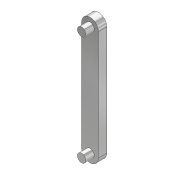
# Autodesk Inventor part: Eslabón 3
Saved by Autodesk Inventor 2021 (Build 250183000, 183)
## iProperties
Created: 2021-10-18
Part Number: Eslabón 3
Material: Steel
Document SubType Name: Modeling
Designer: Usuario
Density: 7.85 g/cm^3
Appearance: Aluminum - Dark
Author: Usuario
Autodesk Inventor part; units mm, degrees
ref_plane "YZ Plane" through (0, 0, 0) normal (1, 0, 0) x (0, 1, 0)
ref_plane "XZ Plane" through (0, 0, 0) normal (0, 1, 0) x (-1, 0, 0)
ref_plane "XY Plane" through (0, 0, 0) normal (0, 0, 1) x (1, 0, 0)
sketch "Sketch1" plane through (0, 0, 0) normal (0, 0, 1) x (1, 0, 0)
  circle A0 centre (0, 0) radius 5
  circle A1 centre (0, 130) radius 5
  circle A2 centre (0, 0) radius 10
  circle A3 centre (0, 130) radius 10
  line L0 (-10, 130) -> (-10, 0)
  line L1 (10, 130) -> (10, 0)
  dimension "d0" = 130
  dimension "d1" = 20
  dimension "d2" = 20
  dimension "d3" = 10
  dimension "d4" = 10
  constraints: 4 centre point, 4 end point, 4 point on circle, 4 tangent, 3 coincident
  measures "d0" distance of point (0, 0) A1.centre
  measures "d1" diameter of A2
  measures "d2" diameter of A3
  measures "d3" diameter of A1
  measures "d4" diameter of A0
extrude "Extrusion1" add sketch "Sketch1" along normal mid plane 10 contours A0 | A1 | A2 | A2 L0 A3 L1 | A3
sketch "Sketch2" plane through (0, 0, 5) normal (0, 0, 1) x (1, 0, 0)
  arc A0 (10, 130) -> (-10, 130) centre (0, 130) ccw construction
  line L0 (-10, 130) -> (-10, 0) construction
  arc A1 (-10, 0) -> (10, 0) centre (0, 0) ccw construction
  line L1 (10, 0) -> (10, 130) construction
  circle A2 centre (0, 130) radius 5
  circle A3 centre (0, 0) radius 5
  dimension "d7" = 10
  dimension "d8" = 10
  constraints: 2 centre point, 2 coincident
  measures "d7" diameter of A2
  measures "d8" diameter of A3
extrude "Extrusion2" add sketch "Sketch2" along normal blind 10
fillet "Fillet1" radius 2 2 edges at (-5, 130, 5) (-5, 0, 5)
body "Solid1"
